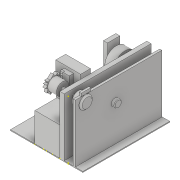
# Autodesk Inventor part: Sujay_tape_roller
Saved by Autodesk Inventor 2019 (Build 230136000, 136)
## iProperties
Created: 2020-03-05
Part Number: Sujay_tape_roller
Material: Generic
Document SubType Name: Modeling
Designer: Abhinav Gupta
Density: 1 g/cm^3
Appearance: Default
Author: Abhinav Gupta
Autodesk Inventor part; units mm, degrees
ref_plane "YZ Plane" through (0, 0, 0) normal (1, 0, 0) x (0, 1, 0)
ref_plane "XZ Plane" through (0, 0, 0) normal (0, 1, 0) x (-1, 0, 0)
ref_plane "XY Plane" through (0, 0, 0) normal (0, 0, 1) x (1, 0, 0)
sketch "Sketch1" plane through (0, 0, 0) normal (0, 0, 1) x (1, 0, 0)
  point P0 (0, 0)
sketch "Sketch2" plane through (0, 0, 0) normal (0, 1, 0) x (-1, 0, 0)
  line L0 (0, 0) -> (200, 0)
  line L1 (200, 0) -> (200, -300)
  line L2 (200, -300) -> (0, -300)
  line L3 (0, -300) -> (0, 0)
  dimension "d0" = 200
  dimension "d1" = 300
  constraints: 8 end point, 2 parallel, 1 horizontal, 1 perpendicular
  measures "d0" distance of L1.end L2.end
  measures "d1" distance of L0.end L1.end
extrude "Extrusion1" add sketch "Sketch2" against normal blind 3
sketch "Sketch3" plane through (0, 0, 0) normal (0, 1, 0) x (1, 0, 0)
  point P0 (0, 0)
sketch "Sketch4" plane through (0, -3, 0) normal (0, -1, 0) x (1, 0, 0)
  point P0 (0, 0)
sketch "Sketch5" plane through (0, 0, 0) normal (0, 1, 0) x (1, 0, 0)
  line L0 (0, 0) -> (-200, 0) projected
  line L1 (-200, 300) -> (0, 300) projected
  line L2 (-14.1271, 0) -> (-14.1271, 300)
  line L3 (-14.1271, 300) -> (-29.1271, 300)
  line L4 (-29.1271, 300) -> (-29.1271, 0)
  line L5 (-29.1271, 0) -> (-14.1271, 0)
  dimension "d4" = 15
  constraints: 8 end point, 2 parallel, 2 point on line, 1 perpendicular, 1 vertical
  measures "d4" distance of L3.end L2.end
extrude "Extrusion2" add sketch "Sketch5" along normal blind 200
sketch "Sketch6" plane through (-29.1271, 0, -300) normal (-1, 0, 0) x (0, 0, 1)
  point P0 (300, 0)
sketch "Sketch7" plane through (-29.1271, 0, -300) normal (-1, 0, 0) x (0, 0, 1)
  circle A0 centre (50.2879, 144.2365) radius 6.0991
  point P0 (300, 0)
  constraints: 1 centre point
extrude "Extrusion3" add sketch "Sketch7" along normal blind 25
sketch "Sketch8" plane through (-54.1271, 144.2365, -249.7121) normal (-1, 0, 0) x (0, 0, 1)
  circle A0 centre (0, 0) radius 39.7089
  point P0 (249.7121, -144.2365)
  constraints: 1 centre point
extrude "Extrusion4" add sketch "Sketch8" along normal blind 30
sketch "Sketch9" plane through (-54.1271, 144.2365, -249.7121) normal (1, 0, 0) x (0, 0, -1)
  point P0 (-249.7121, -144.2365)
sketch "Sketch10" plane through (-84.1271, 144.2365, -249.7121) normal (-1, 0, 0) x (0, 0, 1)
  circle A0 centre (0, 0) radius 6.0991
  point P0 (249.7121, -144.2365)
  constraints: 1 centre point
extrude "Extrusion5" add sketch "Sketch10" along normal blind 30
sketch "Sketch11" plane through (0, 200, 0) normal (0, 1, 0) x (1, 0, 0)
  point P0 (0, 0)
sketch "Sketch12" plane through (-29.1271, 0, -300) normal (-1, 0, 0) x (0, 0, 1)
  point P0 (300, 0)
sketch "Sketch13" plane through (-200, -3, 0) normal (0, 0, 1) x (1, 0, 0)
  point P0 (200, 3)
sketch "Sketch14" plane through (-29.1271, 0, -300) normal (-1, 0, 0) x (0, 0, 1)
  line L0 (50.3622, 144.3107) -> (163.0211, 144.3107)
  line L1 (50.3622, 104.2542) -> (163.0211, 104.2542)
  circle A0 centre (163.0211, 125.713) radius 4.2918
  point P0 (300, 0)
  constraints: 4 end point, 2 horizontal, 1 centre point
extrude "Extrusion6" add sketch "Sketch14" along normal blind 25.95
sketch "Sketch15" plane through (-55.0771, 125.713, -136.9789) normal (-1, 0, 0) x (0, 0, 1)
  circle A0 centre (-112.7332, 18.5235) radius 39.7089 projected
  line L0 (-112.7332, -21.1854) -> (-1.7882, -21.1854)
  circle A1 centre (0, 0) radius 21.9334
  point P0 (136.9789, -125.713)
  constraints: 2 end point, 2 horizontal, 1 centre point, 1 vertical alignment, 1 other
extrude "Extrusion7" add sketch "Sketch15" along normal blind 4 contours A1
sketch "Sketch16" plane through (-200, -3, 0) normal (0, 0, 1) x (1, 0, 0)
  point P0 (200, 3)
sketch "Sketch17" plane through (-59.0771, 125.713, -136.9789) normal (-1, 0, 0) x (0, 0, 1)
  circle A0 centre (0, 0) radius 13.5
  point P0 (136.9789, -125.713)
  dimension "d17" = 27
  constraints: 1 centre point
  measures "d17" diameter of A0
extrude "Extrusion8" add sketch "Sketch17" along normal blind 22
sketch "Sketch18" plane through (-200, -3, 0) normal (0, 0, 1) x (1, 0, 0)
  point P0 (200, 3)
sketch "Sketch19" plane through (-81.0771, 125.713, -136.9789) normal (-1, 0, 0) x (0, 0, 1)
  circle A0 centre (0, 0) radius 4.2918 projected
  circle A1 centre (0, 0) radius 21.9334
  point P0 (136.9789, -125.713)
  constraints: 1 centre point, 1 coincident
extrude "Extrusion9" add sketch "Sketch19" along normal blind 4
sketch "Sketch20" plane through (-200, -3, 0) normal (0, 0, 1) x (1, 0, 0)
  point P0 (200, 3)
sketch "Sketch21" plane through (-29.1271, 0, -300) normal (-1, 0, 0) x (0, 0, 1)
  circle A0 centre (163.0211, 80.2918) radius 4.5521
  point P0 (300, 0)
  constraints: 1 centre point
extrude "Extrusion10" add sketch "Sketch21" along normal blind 25.95
sketch "Sketch22" plane through (-55.0771, 80.2918, -136.9789) normal (-1, 0, 0) x (0, 0, 1)
  circle A0 centre (0, 0) radius 4.5521 projected
  circle A1 centre (0, 0) radius 22.9164
  point P0 (136.9789, -80.2918)
  constraints: 1 centre point, 1 coincident
extrude "Extrusion11" add sketch "Sketch22" along normal blind 30
sketch "Sketch23" plane through (-85.0771, 80.2918, -136.9789) normal (-1, 0, 0) x (0, 0, 1)
  circle A0 centre (0, 0) radius 4.5521
  point P0 (136.9789, -80.2918)
  constraints: 1 centre point
extrude "Extrusion12" add sketch "Sketch23" along normal blind 30
sketch "Sketch24" plane through (-85.0771, 125.713, -136.9789) normal (-1, 0, 0) x (0, 0, 1)
  circle A0 centre (0, 0) radius 4.2918 projected
  circle A1 centre (0, 0) radius 4.2918
  point P0 (136.9789, -125.713)
  constraints: 1 centre point, 1 coincident
extrude "Extrusion13" add sketch "Sketch24" along normal blind 30
sketch "Sketch25" plane through (-29.1271, 0, -300) normal (-1, 0, 0) x (0, 0, 1)
  circle A0 centre (163.0211, 125.713) radius 21.9334 projected
  line L0 (163.0211, 103.7796) -> (227.4838, 103.7796)
  line L1 (195.2525, 103.7796) -> (227.4838, 103.7796)
  line L2 (227.4838, 103.7796) -> (227.4838, 145.2305)
  line L3 (227.4838, 145.2305) -> (195.2525, 145.2305)
  line L4 (195.2525, 145.2305) -> (195.2525, 103.7796)
  point P0 (300, 0)
  constraints: 10 end point, 2 horizontal, 2 parallel, 1 collinear, 1 midpoint, 1 perpendicular, 1 vertical alignment, 1 other
extrude "Extrusion14" add sketch "Sketch25" along normal blind 85 contours L4 L3 L2 L0
sketch "Sketch26" plane through (-29.1271, 103.7796, -72.5162) normal (0, 0, 1) x (1, 0, 0)
  line L0 (0, -103.7796) -> (0, 96.2204) projected
  line L1 (0, -3.7796) -> (-85.7953, -3.7796)
  line L2 (-85.7953, -3.7796) -> (-85.7953, -103.7796)
  line L3 (-85.7953, -103.7796) -> (0, -103.7796)
  line L4 (0, -103.7796) -> (0, -3.7796)
  point P0 (29.1271, -103.7796)
  constraints: 8 end point, 2 parallel, 2 perpendicular, 1 midpoint
extrude "Extrusion15" add sketch "Sketch26" against normal blind 33
sketch "Sketch27" plane through (-29.1271, 103.7796, -72.5162) normal (0, 0, 1) x (1, 0, 0)
  line L0 (-85.7953, -3.7796) -> (0, -3.7796) projected
  line L1 (-85.7953, -3.7796) -> (-85.7953, -103.7796)
  line L2 (-85.7953, -103.7796) -> (0, -103.7796)
  line L3 (0, -103.7796) -> (0, -3.7796)
  line L4 (0, -3.7796) -> (-85.7953, -3.7796)
  point P0 (29.1271, -103.7796)
  constraints: 8 end point, 2 parallel, 1 perpendicular, 1 vertical
extrude "Extrusion16" add sketch "Sketch27" along normal blind 73
sketch "Sketch28" plane through (-29.1271, 145.2305, -72.5162) normal (0, 1, 0) x (1, 0, 0)
  line L0 (0.0501, 33) -> (-85.7953, 33)
  line L1 (-85.7953, 33) -> (-85.7953, -1.0178)
  line L2 (-85.7953, -1.0178) -> (0.0501, -1.0178)
  line L3 (0.0501, -1.0178) -> (0.0501, 33)
  point P0 (29.1271, -72.5162)
  constraints: 8 end point, 2 parallel, 1 horizontal, 1 perpendicular
extrude "Extrusion17" add sketch "Sketch28" along normal blind 70
sketch "Sketch29" plane through (-114.9224, 145.2305, -71.4984) normal (0, 0, 1) x (1, 0, 0)
  line L0 (29.8453, 2.4159) -> (29.8453, -41.4509) projected
  line L1 (29.8453, -32.914) -> (29.8453, 60.4608)
  line L2 (29.8453, 60.4608) -> (61.5654, 60.4608)
  line L3 (61.5654, 60.4608) -> (61.5654, -32.914)
  line L4 (61.5654, -32.914) -> (29.8453, -32.914)
  point P0 (114.9224, -145.2305)
  constraints: 8 end point, 2 parallel, 1 collinear, 1 perpendicular, 1 point on line
extrude "Extrusion18" add sketch "Sketch29" along normal blind 15
sketch "Sketch30" plane through (-200, -3, 0) normal (0, 0, 1) x (1, 0, 0)
  point P0 (200, 3)
sketch "Sketch31" plane through (-29.1271, 0, -300) normal (-1, 0, 0) x (0, 0, 1)
  circle A0 centre (265.7359, 178.119) radius 5.4387
  point P0 (300, 0)
  constraints: 1 centre point
extrude "Extrusion19" add sketch "Sketch31" along normal blind 25
sketch "Sketch32" plane through (-54.1271, 178.119, -34.2641) normal (-1, 0, 0) x (0, 0, 1)
  circle A0 centre (0, 0) radius 21.2167
  point P0 (34.2641, -178.119)
  constraints: 1 centre point
extrude "Extrusion20" add sketch "Sketch32" along normal blind 30
sketch "Sketch33" plane through (-29.1271, 0, -300) normal (-1, 0, 0) x (0, 0, 1)
  circle A0 centre (265.7359, 178.119) radius 5.4387 projected
  circle A1 centre (265.7359, 178.119) radius 5.4387
  point P0 (300, 0)
  constraints: 1 centre point, 1 coincident
extrude "Extrusion21" add sketch "Sketch33" against normal blind 30
sketch "Sketch34" plane through (0.8729, 178.119, -34.2641) normal (1, 0, 0) x (0, 0, -1)
  circle A0 centre (0, 0) radius 22.1573
  point P0 (-34.2641, -178.119)
  constraints: 1 centre point
extrude "Extrusion22" add sketch "Sketch34" along normal blind 30
chamfer "Chamfer1" distance 5 angle 45 1 edges at (30.8729, 178.119, -12.1068) measured on face at (30.8729, 173.2213, -28.7358)
sketch "Sketch35" plane through (-114.9224, 0, -105.5162) normal (-1, 0, 0) x (0, 0, 1)
  point P0 (105.5162, 0)
sketch "Sketch36" plane through (-85.0771, 112.3165, -71.4984) normal (-1, 0, 0) x (0, 0, 1)
  line L0 (8.4353, 93.1907) -> (8.4353, 0.4364)
  line L1 (8.4353, 93.1907) -> (14.7034, 87.6835)
  line L2 (71.4984, 87.6835) -> (-228.5016, 87.6835) projected
  line L3 (8.4353, 80.5494) -> (14.7034, 75.0422)
  line L4 (14.7034, 75.0422) -> (8.4353, 67.9081)
  line L5 (14.7034, 62.4009) -> (8.4353, 57.7934)
  line L6 (14.7034, 49.2661) -> (8.4353, 42.132)
  line L7 (15, 93.3748) -> (15, 0) projected
  line L8 (15, 36.3642) -> (8.4353, 28.8925)
  line L9 (15, 23.1247) -> (8.4353, 15.653)
  line L10 (15, 9.8852) -> (8.4353, -1.589)
  line L11 (8.4353, -1.589) -> (8.4353, 80.5494)
  line L12 (8.4353, 80.5494) -> (14.7034, 87.6835)
  line L13 (8.4353, 67.9081) -> (14.7034, 62.4009)
  line L14 (8.4353, 57.7934) -> (14.7034, 49.2661)
  line L15 (8.4353, 42.132) -> (15, 36.3642)
  line L16 (8.4353, 28.8925) -> (15, 23.1247)
  line L17 (8.4353, 15.653) -> (15, 9.8852)
  point P0 (71.4984, -112.3165)
  constraints: 30 end point, 8 parallel, 4 point on line, 3 perpendicular, 1 vertical, 10 other
extrude "Extrusion23" cut sketch "Sketch36" against normal blind 10 contours L7 L16 L8 | L7 L17 L9
sketch "Sketch37" plane through (-85.0771, 112.3165, -71.4984) normal (-1, 0, 0) x (0, 0, 1)
  line L0 (15, 23.1247) -> (8.4353, 28.8925) projected
  line L1 (8.4353, 28.8925) -> (8.4353, 93.3748)
  line L2 (0, 93.3748) -> (15, 93.3748) projected
  line L3 (15, 36.4676) -> (8.4353, 42.3055)
  line L4 (15, 93.3748) -> (15, 36.3642) projected
  line L5 (15, 49.6876) -> (8.4353, 42.3055)
  point P0 (71.4984, -112.3165)
  constraints: 6 end point, 3 point on line, 1 vertical
extrude "Extrusion24" cut sketch "Sketch37" against normal blind 10 contours L5 L4 L3
sketch "Sketch38" plane through (-75.0771, 112.3165, -71.4984) normal (-1, 0, 0) x (0, 0, 1)
  point P0 (71.4984, -112.3165)
sketch "Sketch39" plane through (-85.0771, 112.3165, -71.4984) normal (-1, 0, 0) x (0, 0, 1)
  line L0 (15, 36.4676) -> (8.4353, 42.3055) projected
  line L1 (8.4353, 42.3055) -> (8.4353, 93.1967)
  line L2 (15, 93.3748) -> (15, 49.6876) projected
  line L3 (15, 49.6876) -> (8.4353, 54.0254)
  line L4 (8.4353, 54.0254) -> (15, 57.8747)
  point P0 (71.4984, -112.3165)
  constraints: 6 end point, 2 point on line, 1 vertical
extrude "Extrusion25" cut sketch "Sketch39" against normal blind 10
sketch "Sketch40" plane through (-85.0771, 112.3165, -71.4984) normal (-1, 0, 0) x (0, 0, 1)
  line L0 (8.4353, 54.0254) -> (15, 57.8747) projected
  line L1 (8.4353, 54.0254) -> (8.4353, 93.3678)
  line L2 (15, 57.8747) -> (8.4353, 62.744)
  line L3 (8.4353, 62.744) -> (15, 66.5984)
  line L4 (15, 93.3748) -> (15, 57.8747) projected
  line L5 (15, 66.5984) -> (15, 57.8747)
  line L6 (15, 57.8747) -> (15, 73.6966)
  line L7 (15, 73.6966) -> (8.4353, 69.8422)
  line L8 (15, 66.5984) -> (8.4353, 69.8422)
  line L9 (15, 73.6966) -> (8.4353, 77.3599)
  line L10 (8.4353, 77.3599) -> (15, 81.2142)
  line L11 (15, 81.2142) -> (8.4353, 84.4581)
  point P0 (71.4984, -112.3165)
  constraints: 20 end point, 6 point on line, 3 parallel, 1 collinear, 1 vertical
extrude "Extrusion26" cut sketch "Sketch40" against normal blind 10 contours L2 L3 L4 | L9 L10 L4
sketch "Sketch41" plane through (-85.0771, 112.3165, -71.4984) normal (-1, 0, 0) x (0, 0, 1)
  line L0 (8.3317, 62.6215) -> (8.3317, 93.4282)
  line L1 (14.9332, 66.3752) -> (8.3317, 70.7762)
  line L2 (14.9332, 73.5268) -> (8.3317, 70.7762)
  line L3 (14.9332, 66.3752) -> (14.9332, 73.5268)
  line L4 (15, 0) -> (15, 93.3748) projected
  point P0 (71.4984, -112.3165)
  constraints: 8 end point, 1 parallel, 1 point on line, 1 vertical
extrude "Extrusion27" cut sketch "Sketch41" against normal blind 10
sketch "Sketch42" plane through (-85.0771, 112.3165, -71.4984) normal (-1, 0, 0) x (0, 0, 1)
  line L0 (8.4353, 77.3599) -> (8.4353, 93.1112)
  line L1 (8.4353, 77.3599) -> (15, 81.2142) projected
  line L2 (15, 81.2142) -> (8.4353, 85.2355)
  line L3 (8.4353, 85.2355) -> (14.7307, 88.1437)
  line L4 (14.7307, 88.1437) -> (8.4353, 93.1112)
  line L5 (15, 0) -> (15, 93.3748) projected
  line L6 (15, 81.2142) -> (15, 93.3748)
  line L7 (15, 93.3748) -> (8.4353, 93.1112)
  point P0 (71.4984, -112.3165)
  constraints: 12 end point, 1 collinear, 1 midpoint, 1 vertical
extrude "Extrusion28" cut sketch "Sketch42" against normal blind 10 contours L3 L4 L7 L5 L2
sketch "Sketch43" plane through (-84.1271, 178.119, -34.2641) normal (-1, 0, 0) x (0, 0, 1)
  circle A0 centre (-1.0607, -0.4892) radius 29.3208
  circle A1 centre (-1.0607, -0.4892) radius 21.2167
  circle A2 centre (0, 0) radius 21.2167 projected
  line L0 (0, 21.2167) -> (0, 28.8124)
  line L1 (12.7354, 16.9693) -> (0.9517, 28.7625)
  line L2 (-22.4478, 0.6705) -> (-28.9025, 4.9737) projected
  line L3 (-21.2161, -0.1506) -> (-28.9025, 4.9737)
  line L4 (-28.9025, 4.9737) -> (-18.6797, 10.0606)
  line L5 (-23.4438, 13.2367) -> (-18.6797, 10.0606)
  line L6 (-23.7911, 13.4683) -> (-16.3937, 13.4683)
  line L7 (-16.3937, 13.4683) -> (-20.4104, 21.5403)
  line L8 (-20.4104, 21.5403) -> (-12.8031, 16.9183)
  line L9 (-12.8031, 16.9183) -> (-12.8087, 26.3752)
  line L10 (-12.8087, 26.3752) -> (-4.3841, 20.7588)
  line L11 (-4.3841, 20.7588) -> (0.9517, 28.7625)
  line L12 (12.7354, 16.9693) -> (22.4916, 16.9751)
  line L13 (22.4916, 16.9751) -> (18.4947, 10.3967)
  line L14 (18.4947, 10.3967) -> (27.7882, 4.7502)
  line L15 (27.7882, 4.7502) -> (22.4916, -3.9674)
  line L16 (22.4916, -3.9674) -> (26.9664, -9.103)
  point P0 (34.2641, -178.119)
  constraints: 32 end point, 5 perpendicular, 3 parallel, 1 centre point, 1 coincident, 1 collinear, 1 horizontal, 1 point on line, 1 vertical, 18 other
extrude "Extrusion29" add sketch "Sketch43" along normal blind 10 contours L13 A2 L12 | L8 A1 L7 | L1 A2 L0 L11 | L10 A2 A1 L9 | A1 L8 A2 L7 | L0 A2 L11 | A1 A2 L9 | L3 L2 L4 A1 | A1 L4 A2 L3
sketch "Sketch44" plane through (-84.1271, 178.119, -34.2641) normal (-1, 0, 0) x (0, 0, 1)
  circle A0 centre (0, 0) radius 28.8198
  circle A1 centre (0, 0) radius 21.2167
  line L0 (-21.2167, 0) -> (-28.8198, 0)
  line L1 (-21.2167, 0) -> (-27.6852, -3.8846)
  line L2 (-22.2343, -7.9277) -> (-28.799, -3.0585) projected
  line L3 (-27.6852, -3.8846) -> (-19.5237, -8.305)
  circle A2 centre (0, 0) radius 21.2167 projected
  line L4 (-19.5237, -8.305) -> (-23.8157, -16.2295)
  line L5 (-23.8157, -16.2295) -> (-13.6657, -16.2295)
  line L6 (-13.6657, -16.2295) -> (-13.6657, -25.3738)
  line L7 (-13.6657, -25.3738) -> (-5.5246, -20.4848)
  line L8 (-5.5246, -20.4848) -> (-0.5219, -28.8151)
  line L9 (-0.5219, -28.8151) -> (3.7116, -20.8895)
  line L10 (3.7116, -20.8895) -> (11.4591, -26.4437)
  line L11 (11.4591, -26.4437) -> (13.6657, -16.2295)
  line L12 (13.6657, -16.2295) -> (23.8157, -16.2295)
  line L13 (23.8157, -16.2295) -> (20.418, -5.7665)
  line L14 (20.418, -5.7665) -> (28.8107, -0.7264)
  line L15 (28.8107, -0.7264) -> (20.5752, 5.1776)
  line L16 (20.5752, 5.1776) -> (27.3054, 9.2194)
  line L17 (27.3054, 9.2194) -> (19.1466, 9.1409)
  point P0 (34.2641, -178.119)
  constraints: 34 end point, 8 point on line, 4 parallel, 4 perpendicular, 1 coincident, 1 horizontal alignment, 22 other
extrude "Extrusion30" add sketch "Sketch44" along normal blind 10 contours L16 A1 L17 | L14 A1 L15 | L12 A1 L13 | A1 L3 L1 | L10 A1 L11 | L4 A1 L5 | L8 A1 L9 | L6 A1 L7
sketch "Sketch45" plane through (-84.1271, 178.119, -34.2641) normal (-1, 0, 0) x (0, 0, 1)
  circle A0 centre (0, 0) radius 5.4387 projected
  circle A1 centre (0, 0) radius 21.2169
  point P0 (34.2641, -178.119)
  constraints: 1 centre point, 1 coincident
extrude "Extrusion31" add sketch "Sketch45" along normal blind 10
sketch "Sketch46" plane through (-114.9224, 145.2305, -56.4984) normal (0, 0, 1) x (1, 0, 0)
  point P0 (114.9224, -145.2305)
sketch "Sketch47" plane through (0, 0, 0) normal (0, 1, 0) x (1, 0, 0)
  line L0 (-105.4778, 226.3985) -> (-91.4918, 226.3985)
  line L1 (-91.4918, 226.3985) -> (-91.4918, 269.522)
  line L2 (-91.4918, 269.522) -> (-105.4778, 269.522)
  line L3 (-105.4778, 269.522) -> (-105.4778, 226.3985)
  point P0 (0, 0)
  constraints: 8 end point, 2 parallel, 1 horizontal, 1 perpendicular
extrude "Extrusion32" add sketch "Sketch47" along normal blind 200
sketch "Sketch48" plane through (0, -3, 0) normal (0, -1, 0) x (1, 0, 0)
  point P0 (0, 0)
sketch "Sketch49" plane through (0, 0, 0) normal (1, 0, 0) x (0, 0, -1)
  line L0 (0, 0) -> (105.5162, 0) projected
  line L1 (0, -3) -> (300, -3) projected
  line L2 (0, 0) -> (300, 0)
  line L3 (300, 0) -> (300, -3)
  line L4 (300, -3) -> (0, -3)
  line L5 (0, -3) -> (0, 0)
  constraints: 8 end point, 2 parallel, 1 horizontal, 1 perpendicular
extrude "Extrusion33" add sketch "Sketch49" along normal blind 50
sketch "Sketch50" plane through (-29.1271, 0, -300) normal (-1, 0, 0) x (0, 0, 1)
  point P0 (300, 0)
sketch "Sketch51" plane through (-115.0771, 125.713, -136.9789) normal (-1, 0, 0) x (0, 0, 1)
  circle A0 centre (0, 0) radius 4.1208
  point P0 (136.9789, -125.713)
  constraints: 1 centre point
extrude "Extrusion34" add sketch "Sketch51" against normal blind 120
sketch "Sketch52" plane through (4.9229, 125.713, -136.9789) normal (1, 0, 0) x (0, 0, -1)
  circle A0 centre (0, 0) radius 12.7925
  point P0 (-136.9789, -125.713)
  constraints: 1 centre point
extrude "Extrusion35" add sketch "Sketch52" along normal blind 30
fillet "Fillet1" radius 2 1 edges at (34.9229, 125.713, -124.1865)
sketch "Sketch53" plane through (0, 0, 0) normal (0, 1, 0) x (1, 0, 0)
  line L0 (-106.2019, 156.618) -> (-98.4456, 156.618)
  line L1 (-98.4456, 156.618) -> (-98.4456, 118.433)
  line L2 (-98.4456, 118.433) -> (-106.2019, 118.433)
  line L3 (-106.2019, 118.433) -> (-106.2019, 156.618)
  point P0 (0, 0)
  constraints: 8 end point, 2 parallel, 1 horizontal, 1 perpendicular
extrude "Extrusion36" add sketch "Sketch53" along normal blind 150
sketch "Sketch54" plane through (-85.0771, 112.3165, -71.4984) normal (-1, 0, 0) x (0, 0, 1)
  point P0 (71.4984, -112.3165)
sketch "Sketch55" plane through (0, 0, 0) normal (0, 1, 0) x (1, 0, 0)
  line L0 (24.1064, 0) -> (16.5398, 0)
  line L1 (16.5398, 0) -> (16.5398, 298.7981)
  line L2 (16.5398, 298.7981) -> (24.1064, 298.7981)
  line L3 (24.1064, 298.7981) -> (24.1064, 0)
  point P0 (0, 0)
  constraints: 8 end point, 2 parallel, 1 horizontal, 1 perpendicular
extrude "Extrusion37" add sketch "Sketch55" along normal blind 200
sketch "Sketch56" plane through (0, 200, 0) normal (0, 1, 0) x (1, 0, 0)
  line L0 (16.5398, 0) -> (16.5398, 298.7981) projected
  line L1 (23.5184, 20.8726) -> (16.5398, 20.8726)
  line L2 (16.5398, 20.8726) -> (16.5398, 54.3863)
  line L3 (16.5398, 54.3863) -> (23.5184, 54.3863)
  line L4 (23.5184, 54.3863) -> (23.5184, 20.8726)
  point P0 (0, 0)
  constraints: 8 end point, 2 parallel, 1 horizontal, 1 perpendicular, 1 point on line
extrude "Extrusion38" add sketch "Sketch56" along normal blind 10
body "Solid1"
